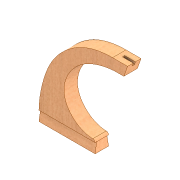
# Autodesk Inventor part: TNS-1-arm
Saved by Autodesk Inventor 2020 (Build 240168000, 168)
## iProperties
Created: 2021-06-28
Part Number: TNS-1-arm
Material: Generic
Document SubType Name: Modeling
Designer: Aidan Lee
Density: 1 g/cm^3
Appearance: Cherry - Natural Low Gloss
Author: Aidan Lee
Autodesk Inventor part; units mm, degrees
ref_plane "XZ Plane" through (0, 0, 0) normal (0, 1, 0) x (-1, 0, 0)
ref_plane "XY Plane" through (0, 0, 0) normal (0, 0, 1) x (1, 0, 0)
sketch "Sketch1" plane through (0, 0, 0) normal (0, 0, 1) x (1, 0, 0)
  line L0 (60, 34) -> (279, 34) construction
  line L1 (279, 34) -> (279, 16) construction
  line L2 (279, 16) -> (60, 16) construction
  line L3 (60, 16) -> (60, 34) construction
  line L4 (158.3401, 144) -> (180.6599, 144)
  line L5 (-98.1271, 119.3914) -> (-155.2055, 119.3914) construction
  line L6 (60, 204.7828) -> (279, 204.7828) construction
  line L7 (279, 204.7828) -> (279, 222.7828) construction
  line L8 (279, 222.7828) -> (60, 222.7828) construction
  line L9 (60, 222.7828) -> (60, 204.7828) construction
  line L10 (158.3401, 94.7828) -> (180.6599, 94.7828) construction
  line L11 (169.5, 144) -> (169.5, 94.7828) construction
  circle A0 centre (169.5, 144.5) radius 4.5 construction
  circle A1 centre (169.5, 94.2828) radius 4.5 construction
  line L12 (165, 140) -> (174, 140) construction
  spline S0 degree 4 poles (60, 34) (60, 50.8003) (67.6192, 82.543) (79.1211, 110.1157) (114.0169, 138.9549) (142.0747, 144) (158.3401, 144) knots 0 0 0 0 0 0.37584 0.62584 1 1 1 1 1
  line L13 (436.9307, -63.7999) -> (436.9307, -111.3151) construction
  line L14 (165.0658, 130) -> (173.4412, 130)
  line L15 (173.4412, 130) -> (178.3964, 144)
  line L16 (178.3964, 144) -> (180.6599, 144)
  line L17 (166.2744, 149) -> (172.7256, 149) construction
  spline S1 degree 4 poles (165.0658, 130) (150.6222, 130) (124.5762, 123.7444) (97.0964, 105.142) (83.3994, 60.1633) (114.2343, 37) (132, 37) knots 0 0 0 0 0 0.366098 0.616098 1 1 1 1 1
  line L18 (158.3401, 94.7828) -> (180.6599, 94.7828) construction
  line L19 (178.3964, 94.7828) -> (180.6599, 94.7828) construction
  line L20 (180.6599, 94.7828) -> (158.3401, 94.7828) construction
  spline S2 degree 4 poles (173.9342, 106.4847) (188.3699, 106.4847) (225.2165, 124.0597) (250.4536, 142.2568) (239.0722, 211.617) (207.7908, 202.4847) knots 0 0 0 0 0 0.376784 1 1 1 1 1 construction
  spline S3 degree 4 poles (279, 204.7828) (275.6992, 148.3745) (255.9313, 132.0927) (229.7092, 97.2581) (180.6599, 94.7828) knots 0 0 0 0 0 1 1 1 1 1 construction
  line L21 (173.9342, 106.4847) -> (158.8804, 106.4847) construction
  line L22 (160.6036, 94.7828) -> (158.3401, 94.7828) construction
  line L23 (158.8804, 106.4847) -> (160.6036, 94.7828) construction
  arc A2 (135, 34) -> (132, 37) centre (132, 34) ccw
  line L24 (135, 34) -> (60, 34)
  point P0 (0, 0)
  point P1 (169.5, 34)
  point P2 (169.5, 204.7828)
  point P3 (93.4315, 204.7828)
  point P4 (169.5, 140)
  point P5 (69.0653, 81.3021)
  point P6 (84.771, 109.712)
  point P7 (114.2865, 133.8506)
  point P8 (169.5, 149)
  point P9 (126.5497, 121.1282)
  point P10 (101.7633, 99.5435)
  point P11 (94.9383, 64.5723)
  point P12 (209.9254, 118.4197)
  point P13 (233.3153, 142.9189)
  point P14 (236.6483, 184.5924)
  point P15 (268.3461, 156.1626)
  point P16 (250.8428, 129.4297)
  point P17 (224.4145, 107.9607)
  dimension "d0" = 18
  dimension "d2" = 219
  dimension "d4" = 16
  dimension "d5" = 60
  dimension "d6" = 110
  dimension "d9" = 9
  dimension "d11" = 10
  dimension "exposed" = 5
  dimension "d13" = 14
  dimension "d23" = 3
  dimension "d43" = 75
  dimension "d48" = 109.5
  constraints: 50 end point, 13 symmetric about line, 8 horizontal, 5 midpoint, 4 parallel, 4 point on circle, 3 centre point, 3 point on line, 3 vertical alignment, 2 tangent, 2 vertical, 1 collinear, 1 perpendicular, 22 other
  measures "d0" distance of L2.end L0.start
  measures "d2" distance of L1.end L2.end
  measures "d4" distance from line of point (0, 0) L2
  measures "d5" horizontal distance of point (0, 0) L2.end
  measures "d6" distance between parallel lines of L0 L4
  measures "d9" diameter of A0
  measures "d11" distance between parallel lines of L12 L14
  measures "exposed" distance between parallel lines of L17 L4
  measures "d13" distance between parallel lines of L4 L14
  measures "d23" radius of A2
  measures "d43" distance of L0.start L24.start
  measures "d48" distance between parallel lines of L11 L3
extrude "Extrusion1" add sketch "Sketch1" along normal blind 18
sketch "Sketch4" plane through (158.3401, 144, 0) normal (0, 1, 0) x (1, 0, 0)
  line L0 (-98.3401, -118.5) -> (120.6599, -118.5) construction
  line L1 (120.6599, -118.5) -> (120.6599, 100.5) construction
  line L2 (120.6599, 100.5) -> (-98.3401, 100.5) construction
  circle A0 centre (11.1599, -9) radius 1
  line L3 (-98.3401, 0) -> (-98.3401, -18) projected
  line L4 (20.0563, 0) -> (20.0563, -18) projected
  point P0 (-158.3401, 0)
  point P1 (11.1599, -118.5)
  point P2 (120.6599, -9)
  point P3 (20.0563, -9)
  dimension "d30" = 219
  dimension "d31" = 219
  dimension "d32" = 2
  dimension "d49" = 109.5
  constraints: 6 end point, 3 midpoint, 2 horizontal alignment, 1 centre point, 1 horizontal, 1 parallel, 1 perpendicular, 1 vertical alignment
  measures "d30" distance of L2.end L0.start
  measures "d31" distance of L0.start L0.end
  measures "d32" diameter of A0
  measures "d49" distance from line of A0.centre L3
extrude "Extrusion5" cut sketch "Sketch4" against normal through all
sketch "Sketch5" plane through (158.3401, 144, 0) normal (0, 1, 0) x (1, 0, 0)
  line L0 (26.7348, -7.5) -> (5.6599, -7.5)
  line L1 (5.6599, -7.5) -> (5.6599, -10.5)
  line L2 (5.6599, -10.5) -> (26.7348, -10.5)
  line L3 (26.7348, -10.5) -> (26.7348, -7.5)
  circle A0 centre (11.1599, -9) radius 1 projected
  line L4 (6.6599, -8.6) -> (15.6599, -8.6) construction
  line L5 (15.6599, -8.6) -> (15.6599, -9.4) construction
  line L6 (15.6599, -9.4) -> (6.6599, -9.4) construction
  line L7 (6.6599, -9.4) -> (6.6599, -8.6) construction
  point P0 (-158.3401, 0)
  point P1 (5.6599, -9)
  point P2 (6.6599, -9)
  point P3 (11.1599, -8.6)
  point P4 (11.1599, -10.5)
  point P5 (11.1599, -7.5)
  dimension "d35" = 3
  dimension "d36" = 9
  dimension "d37" = 0.8
  dimension "d41" = 1
  constraints: 16 end point, 4 parallel, 3 midpoint, 2 horizontal, 2 horizontal alignment, 2 perpendicular, 1 vertical alignment
  measures "d35" distance of L0.end L1.end
  measures "d36" distance of L4.start L4.end
  measures "d37" distance of L4.end L5.end
  measures "d41" distance between parallel lines of L1 L7
extrude "Extrusion6" cut sketch "Sketch5" against normal blind 4 contours L3 L2 L1 L0 | A0
ref_plane "Work Plane3" through (60, 34, 18) normal (1, 0, 0) x (0, 1, 0)
sketch "Sketch6" plane through (60, 34, 18) normal (1, 0, 0) x (0, 1, 0)
  line L0 (-13, -18) -> (-13, 0)
  line L1 (0, -18) -> (0, 0) projected
  line L2 (-13, -18) -> (0, -15.8012)
  line L3 (0, -18) -> (0, 0) projected
  line L4 (0, -15.8012) -> (-9.0304, -15.8012) construction
  line L5 (-15.1424, -9) -> (-18.4796, -9) construction
  line L6 (-13, 0) -> (0, -2.1988)
  point P0 (-34, -18)
  point P1 (-16.811, -9)
  point P2 (-13, -9)
  dimension "d44" = 13
  dimension "d45" = 9.6
  constraints: 10 end point, 3 horizontal alignment, 2 horizontal, 2 midpoint, 1 point on line, 1 symmetric about line, 1 vertical
  measures "d44" distance between parallel lines of L1 L0
  measures "d45" angle of L4 L2
extrude "Extrusion7" add sketch "Sketch6" along normal up to surface (75 mm away)
body "Solid1"
